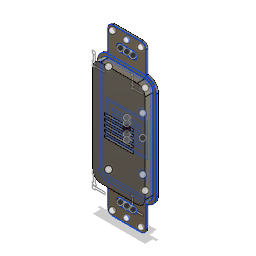
Thermostat cover (Autodesk Fusion 360 design; units mm, degrees)
Autodesk Fusion 360 part; units mm, degrees
sketch "Sketch1" plane through (0, 0, 0) normal (0, 0, 1) x (1, 0, 0) in component "Main plate"
  line L0 (12, -33) -> (12, -49)
  line L1 (-11.5, -33) -> (11.5, -33)
  line L2 (11.5, 33) -> (-11.5, 33)
  line L3 (-9, 52) -> (9, 52)
  line L4 (-12, 33) -> (-12, 49)
  line L5 (16.5, -28) -> (16.5, 28)
  line L6 (-12, -49) -> (-12, -33)
  circle A0 centre (0, -48.5) radius 1.35
  circle A1 centre (0, 48.5) radius 1.35
  line L7 (9, -52) -> (-9, -52)
  line L8 (12, 49) -> (12, 33)
  arc A2 (-11.5, 33) -> (-16.5, 28) centre (-11.5, 28) ccw
  line L9 (-16.5, 28) -> (-16.5, -28)
  arc A3 (16.5, 28) -> (11.5, 33) centre (11.5, 28) ccw
  arc A4 (11.5, -33) -> (16.5, -28) centre (11.5, -28) ccw
  arc A5 (-16.5, -28) -> (-11.5, -33) centre (-11.5, -28) ccw
  arc A6 (-12, -49) -> (-9, -52) centre (-9, -49) ccw
  arc A7 (9, -52) -> (12, -49) centre (9, -49) ccw
  arc A8 (-9, 52) -> (-12, 49) centre (-9, 49) ccw
  arc A9 (12, 49) -> (9, 52) centre (9, 49) ccw
  line L10 (-11.5, -35) -> (11.5, -35)
  arc A10 (11.5, -35) -> (18.5, -28) centre (11.5, -28) ccw
  line L11 (18.5, -28) -> (18.5, 28)
  arc A11 (18.5, 28) -> (11.5, 35) centre (11.5, 28) ccw
  line L12 (11.5, 35) -> (-11.5, 35)
  arc A12 (-11.5, 35) -> (-18.5, 28) centre (-11.5, 28) ccw
  line L13 (-18.5, 28) -> (-18.5, -28)
  arc A13 (-18.5, -28) -> (-11.5, -35) centre (-11.5, -28) ccw
  line L14 (-4, 39.75) -> (4, 39.75)
  arc A14 (4, 39.75) -> (4, 44.25) centre (4, 42) ccw
  line L15 (4, 44.25) -> (-4, 44.25)
  arc A15 (-4, 44.25) -> (-4, 39.75) centre (-4, 42) ccw
  line L16 (-4, 42) -> (4, 42) construction
  line L17 (-4, -42) -> (4, -42) construction
  arc A16 (4, -44.25) -> (4, -39.75) centre (4, -42) ccw
  line L18 (-4, -44.25) -> (4, -44.25)
  arc A17 (-4, -39.75) -> (-4, -44.25) centre (-4, -42) ccw
  line L19 (4, -39.75) -> (-4, -39.75)
  line L20 (-11.5, -31.5) -> (11.5, -31.5)
  arc A18 (11.5, -31.5) -> (15, -28) centre (11.5, -28) ccw
  line L21 (15, -28) -> (15, 28)
  arc A19 (15, 28) -> (11.5, 31.5) centre (11.5, 28) ccw
  line L22 (11.5, 31.5) -> (-11.5, 31.5)
  arc A20 (-11.5, 31.5) -> (-15, 28) centre (-11.5, 28) ccw
  line L23 (-15, 28) -> (-15, -28)
  arc A21 (-15, -28) -> (-11.5, -31.5) centre (-11.5, -28) ccw
  line L24 (9, -0.75) -> (-9, -0.75)
  line L25 (-9, -0.75) -> (-9, 0.75)
  line L26 (-9, 0.75) -> (9, 0.75)
  line L27 (9, 0.75) -> (9, -0.75)
  line L28 (9, 3.75) -> (9, 2.25)
  line L29 (9, 2.25) -> (-9, 2.25)
  line L30 (-9, 2.25) -> (-9, 3.75)
  line L31 (-9, 3.75) -> (9, 3.75)
  line L32 (-9, 5.25) -> (-9, 6.75)
  line L33 (-9, 6.75) -> (9, 6.75)
  line L34 (9, 5.25) -> (-9, 5.25)
  line L35 (9, 6.75) -> (9, 5.25)
  line L36 (-9, -2.25) -> (9, -2.25)
  line L37 (9, -2.25) -> (9, -3.75)
  line L38 (-9, -3.75) -> (-9, -2.25)
  line L39 (9, -3.75) -> (-9, -3.75)
  line L40 (9, -5.25) -> (9, -6.75)
  line L41 (-9, -5.25) -> (9, -5.25)
  line L42 (-9, -6.75) -> (-9, -5.25)
  line L43 (9, -6.75) -> (-9, -6.75)
  line L44 (12, -9.5) -> (-12, -9.5)
  line L45 (-12, -9.5) -> (-12, 9.5)
  line L46 (-12, 9.5) -> (12, 9.5)
  line L47 (12, 9.5) -> (12, -9.5)
  line L48 (13, -10.5) -> (-13, -10.5)
  line L49 (-13, -10.5) -> (-13, 10.5)
  line L50 (-13, 10.5) -> (13, 10.5)
  line L51 (13, 10.5) -> (13, -10.5)
  circle A22 centre (10, 13.5) radius 1.45
  circle A23 centre (10, -20) radius 1.45
  circle A24 centre (10, 13.5) radius 2.45
  circle A25 centre (10, -20) radius 2.45
  point P0 (10, 0)
  point P1 (10, 0)
  point P2 (0, 42)
  point P3 (0, -42)
  point P4 (0, 3)
  point P5 (0, 3)
  point P6 (0, 3)
  point P7 (0, 3)
  point P8 (0, 6)
  point P9 (0, 6)
  point P10 (0, 6)
  point P11 (0, 6)
  point P12 (0, -3)
  point P13 (0, -3)
  point P14 (0, -3)
  point P15 (0, -3)
  point P16 (0, -6)
  point P17 (0, -6)
  point P18 (0, -6)
  point P19 (0, -6)
  point P20 (10, 0)
  dimension "d15" = 5
  dimension "d16" = 5
  dimension "d17" = 3
  dimension "d18" = 3
  dimension "d19" = 3
  dimension "d20" = 3
  dimension "d26" = 4.5
  dimension "d27" = 4.5
  dimension "d54" = 2.9
  dimension "d55" = 2.9
  dimension "d56" = 1
  dimension "d57" = 1
  constraint horizontal L1
  constraint vertical L5
  constraint horizontal L2
  constraint vertical L9
  constraint horizontal L3
  constraint vertical L8
  constraint horizontal L7
  constraint vertical L6
  constraint coincident L6.end L1
  constraint coincident L4.start L2
  constraint collinear L4 L6
  constraint coincident L8.end L2
  constraint coincident L0.start L1
  constraint collinear L0 L8
  constraint coincident P20 P0
  constraint tangent L2 A2
  constraint tangent A2 L9
  constraint tangent L2 A3
  constraint tangent L5 A3
  constraint tangent L5 A4
  constraint tangent L1 A4
  constraint equal A3 A4
  constraint tangent L9 A5
  constraint tangent L1 A5
  constraint equal A3 A5
  constraint tangent L6 A6
  constraint tangent L7 A6
  constraint tangent L7 A7
  constraint tangent L0 A7
  constraint tangent L4 A8
  constraint tangent L3 A8
  constraint tangent L3 A9
  constraint tangent L8 A9
  constraint tangent L14 A14
  constraint tangent A14 L15
  constraint parallel L14 L15
  constraint tangent L15 A15
  constraint tangent L14 A15
  constraint horizontal L16
  constraint midpoint L16 P2
  constraint tangent A16 L18
  constraint tangent A16 L19
  constraint parallel L18 L19
  constraint tangent A17 L19
  constraint tangent L18 A17
  constraint horizontal L17
  constraint midpoint P3 L17
  constraint perpendicular L24 L25
  constraint parallel L24 L26
  constraint parallel L25 L27
  constraint horizontal L24
  constraint coincident P7 P6
  constraint perpendicular L29 L30
  constraint parallel L29 L31
  constraint parallel L28 L30
  constraint horizontal L29
  constraint coincident P11 P10
  constraint perpendicular L32 L34
  constraint parallel L33 L34
  constraint parallel L32 L35
  constraint horizontal L34
  constraint coincident P15 P14
  constraint perpendicular L38 L39
  constraint parallel L36 L39
  constraint parallel L37 L38
  constraint horizontal L39
  constraint coincident P19 P18
  constraint perpendicular L42 L43
  constraint parallel L41 L43
  constraint parallel L40 L42
  constraint horizontal L43
  constraint perpendicular L44 L45
  constraint parallel L44 L46
  constraint parallel L45 L47
  constraint horizontal L44
  constraint parallel L1 L10
  constraint concentric A4 A10
  constraint parallel L5 L11
  constraint concentric A3 A11
  constraint parallel L2 L12
  constraint concentric A2 A12
  constraint parallel L9 L13
  constraint concentric A5 A13
  constraint tangent L10 A13
  constraint tangent L10 A10
  constraint tangent A11 L12
  constraint tangent A10 L11
  constraint tangent A12 L13
  constraint tangent L11 A11
  constraint tangent L12 A12
  constraint tangent L13 A13
  constraint parallel L1 L20
  constraint concentric A4 A18
  constraint parallel L5 L21
  constraint concentric A3 A19
  constraint parallel L2 L22
  constraint concentric A2 A20
  constraint parallel L9 L23
  constraint concentric A5 A21
  constraint tangent A19 L22
  constraint tangent L20 A21
  constraint tangent L20 A18
  constraint tangent A18 L21
  constraint tangent L22 A20
  constraint tangent L21 A19
  constraint tangent A20 L23
  constraint tangent L23 A21
  constraint parallel L44 L48
  constraint parallel L45 L49
  constraint parallel L46 L50
  constraint parallel L47 L51
  measures "d15" radius of A2
  measures "d16" radius of A3
  measures "d17" radius of A6
  measures "d18" radius of A7
  measures "d19" radius of A8
  measures "d20" radius of A9
  measures "d26" diameter of A14
  measures "d27" diameter of A16
  measures "d54" diameter of A22
  measures "d55" diameter of A23
extrude "Extrude1" add sketch "Sketch1" along normal blind 5 contours L1 L2 L5 A2 L9 A3 A4 A5 | L20 A18 L21 A19 L22 A20 L23 A21 | L24 L25 L26 L27 | L28 L29 L30 L31 | L32 L33 L34 L35 | L36 L37 L38 L39 | L40 L41 L42 L43 | L44 L45 L46 L47 | L48 L49 L50 L51 | A22 | A23 | A24 | A25 makes body 1 in component "Main plate"
extrude "Extrude2" add sketch "Sketch1" against normal blind 1.5 separate body contours L0 L6 L7 A6 A7 L10 A10 A13 | L10 A10 L11 A11 L12 A12 L13 A13 | L3 L4 L8 A8 A9 A11 L12 A12 | L14 A14 L15 A15 | A16 L18 A17 L19 makes body 2 in component "Main plate"
extrude "Extrude3" cut sketch "Sketch1" against normal through all contours L14 A14 L15 A15 bodies 2 in component "Main plate"
extrude "Extrude4" cut sketch "Sketch1" against normal through all contours A16 L18 A17 L19 bodies 2 in component "Main plate"
extrude "Extrude5" add sketch "Sketch1" against normal blind 1.5 contours L1 L2 L5 A2 L9 A3 A4 A5 | L20 A18 L21 A19 L22 A20 L23 A21 | L24 L25 L26 L27 | L28 L29 L30 L31 | L32 L33 L34 L35 | L36 L37 L38 L39 | L40 L41 L42 L43 | L44 L45 L46 L47 | L48 L49 L50 L51 | A22 | A23 | A24 | A25 bodies 1 2 in component "Main plate"
extrude "Extrude6" cut sketch "Sketch1" along normal blind 3.5 contours L20 A18 L21 A19 L22 A20 L23 A21 | L24 L25 L26 L27 | L28 L29 L30 L31 | L32 L33 L34 L35 | L36 L37 L38 L39 | L40 L41 L42 L43 | L44 L45 L46 L47 | L48 L49 L50 L51 | A22 | A23 | A24 | A25 bodies 1 in component "Main plate"
extrude "Extrude7" add sketch "Sketch1" along normal blind 3.5 separate body contours L20 A18 L21 A19 L22 A20 L23 A21 | L24 L25 L26 L27 | L28 L29 L30 L31 | L32 L33 L34 L35 | L36 L37 L38 L39 | L40 L41 L42 L43 | L44 L45 L46 L47 | L48 L49 L50 L51 | A22 | A23 | A24 | A25 makes body 3 in component "Main plate"
extrude "Extrude8" add sketch "Sketch1" against normal blind 1.5 contours L20 A18 L21 A19 L22 A20 L23 A21 | L24 L25 L26 L27 | L28 L29 L30 L31 | L32 L33 L34 L35 | L36 L37 L38 L39 | L40 L41 L42 L43 | L44 L45 L46 L47 | L48 L49 L50 L51 | A22 | A23 | A24 | A25 bodies 3 in component "Main plate"
combine "Combine1" operation cut target body 1 tool bodies 3 in component "Main plate"
extrude "Extrude9" add sketch "Sketch1" along normal blind 13 separate body contours L24 L25 L26 L27 | L28 L29 L30 L31 | L32 L33 L34 L35 | L36 L37 L38 L39 | L40 L41 L42 L43 makes body 4 at (3, -0.75, 4.3333) makes body 5 at (-3, -2.25, 4.3333) makes body 6 at (3, 2.25, 4.3333) makes body 7 at (3, -6.75, 4.3333) makes body 8 at (-3, 6.75, 4.3333) in component "Main plate"
combine "Combine2" operation cut target body 1 tool bodies 8 6 4 5 7 in component "Main plate"
extrude "Extrude10" add sketch "Sketch1" along normal blind 4 contours L48 L49 L50 L51 bodies 1 in component "Main plate"
extrude "Extrude11" add 1 faces at (-4, -10.1667, 0) along direction (0, 0, -1) blind 4.5 on bodies 1 bodies 1 in component "Main plate"
extrude "Extrude12" add sketch "Sketch1" along normal blind 3.5 separate body contours A24 makes body 9 in component "Main plate"
extrude "Extrude13" add sketch "Sketch1" against normal blind 6.5 contours A24 bodies 9 in component "Main plate"
extrude "Extrude14" add sketch "Sketch1" along normal blind 3.5 separate body contours A25 makes body 10 in component "Main plate"
extrude "Extrude15" add sketch "Sketch1" against normal blind 6.5 contours A25 bodies 10 in component "Main plate"
combine "Combine3" operation add target body 1 tool bodies 9 10 in component "Main plate"
component "Main plate" placed x (1, 0, 0) y (0, 1, 0) z (0, 0, 1) at (0, 0, 0)
named bodies: "Plate", "Side and wings"
